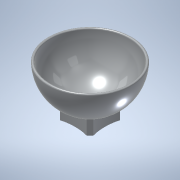
# Autodesk Inventor part: Bowlcup
Saved by Autodesk Inventor 2021 (Build 250183000, 183)
## iProperties
Created: 2013-08-09
Part Number: Bowlcup
Material: Glass
Document SubType Name: Modeling
Designer: Kenan K
Density: 1 g/cm^3
Appearance: Clear
Author: Kenan K
Autodesk Inventor part; units mm, degrees
ref_plane "YZ Plane" through (0, 0, 0) normal (1, 0, 0) x (0, 1, 0)
ref_plane "XY Plane" through (0, 0, 0) normal (0, 0, 1) x (1, 0, 0)
sketch "Sketch1" plane through (0, 0, 0) normal (0, 0, 1) x (1, 0, 0)
  line L0 (0, 36) -> (4, 40)
  line L1 (0, 4) -> (4, 0)
  line L2 (40, 4) -> (36, 0)
  line L3 (36, 40) -> (40, 36)
  arc A0 (0, 4) -> (0, 36) centre (-57.8273, 20) ccw
  arc A1 (4, 40) -> (36, 40) centre (20, 97.8273) ccw
  arc A2 (36, 0) -> (4, 0) centre (20, -57.8273) ccw
  arc A3 (40, 36) -> (40, 4) centre (97.8273, 20) ccw
  point P0 (0, 0)
  point P1 (40, 40)
  point P2 (40, 0)
  point P3 (0, 40)
  dimension "d0" = 40
  dimension "d1" = 40
  dimension "d2" = 4
  dimension "d3" = 4
  dimension "d4" = 4
  dimension "d5" = 4
  dimension "d6" = 4
  dimension "d7" = 4
  dimension "d8" = 4
  dimension "d9" = 4
  dimension "d10" = 60
  dimension "d11" = 60
  dimension "d12" = 60
  dimension "d13" = 60
  constraints: 8 end point, 8 point on circle, 4 centre point
  measures "d0" distance of point (0, 40) point (40, 40)
  measures "d1" distance of point (40, 40) point (40, 0)
  measures "d2" distance of L0.start point (0, 40)
  measures "d3" distance of L0.end point (0, 40)
  measures "d4" distance of L1.start point (0, 0)
  measures "d5" distance of L1.end point (0, 0)
  measures "d6" distance of L2.start point (40, 0)
  measures "d7" distance of L2.end point (40, 0)
  measures "d8" distance of L3.start point (40, 40)
  measures "d9" distance of L3.end point (40, 40)
  measures "d10" radius of A0
  measures "d11" radius of A1
  measures "d12" radius of A2
  measures "d13" radius of A3
extrude "Extrusion1" add sketch "Sketch1" along normal blind 20
sketch "Sketch2" plane through (0, 0, 0) normal (0, 0, -1) x (-1, 0, 0)
  arc A0 (-34.5, 36) -> (-37.5, 36) centre (-36, 36) ccw
  line L0 (-37.5, 36) -> (-34.5, 36)
  point P0 (0, 0)
  dimension "d16" = 3
  constraints: 2 end point, 2 point on circle, 1 centre point, 1 horizontal
  measures "d16" diameter of A0
revolve "Revolution1" add sketch "Sketch2" angle 360 about axis through (37.5, 36, 0) along (-1, 0, 0)
pattern_linear "Rectangular Pattern1" count 2 spacing 32 along (-1, 0, 0) count 2 spacing 32 along (0, -1, 0) of "Revolution1"
ref_plane "Work Plane1" through (0, 20, 0) normal (0, 1, 0) x (-1, 0, 0)
sketch "Sketch3" plane through (0, 20, 0) normal (0, 1, 0) x (-1, 0, 0)
  line L0 (0, 0) -> (0, 20) projected
  line L1 (-40, 0) -> (-40, 20) projected
  arc A0 (-20, 10) -> (30, 60) centre (-20, 60) ccw
  arc A1 (-20, 13) -> (27, 60) centre (-20, 60) ccw
  line L2 (-20, 10) -> (-20, 13)
  line L3 (27, 60) -> (30, 60)
  dimension "d41" = 3
  constraints: 5 point on circle, 4 end point, 2 centre point, 1 perpendicular, 2 other
  measures "d41" distance of L3.end L3.start
revolve "Revolution3" add sketch "Sketch3" angle 360 about axis through (20, 20, 10) along (0, 0, 1)
sketch "Sketch4" plane through (20, 20, 60) normal (0, 0, 1) x (1, 0, 0)
  circle A0 centre (0, 0) radius 47 projected
  circle A1 centre (0, 0) radius 50 projected
  arc A2 (47, 0) -> (-47, 0) centre (0, 0) ccw
  line L0 (0, 0) -> (47, 0)
  line L1 (-47, 0) -> (0, 0)
  point P0 (-20, -20)
  constraints: 4 end point, 2 point on circle, 1 centre point, 1 coincident, 1 collinear, 1 concentric, 1 horizontal
revolve "Revolution4" cut sketch "Sketch4" angle 360 about axis through (20, 20, 60) along (1, 0, 0) picked at (-27.5005, 14.6993) contours L0 L1 A0
fillet "Fillet1" radius 1.5 2 edges at (70, 20, 60) (67, 20, 60)
equation "\"d3\" = d2"
equation "\"d4\" = d2"
equation "\"d5\" = d4"
equation "\"d6\" = d2"
equation "\"d7\" = d6"
equation "\"d8\" = d2"
equation "\"d9\" = d8"
equation "\"d12\" = d10"
equation "\"d13\" = d10"
body "Solid1"
